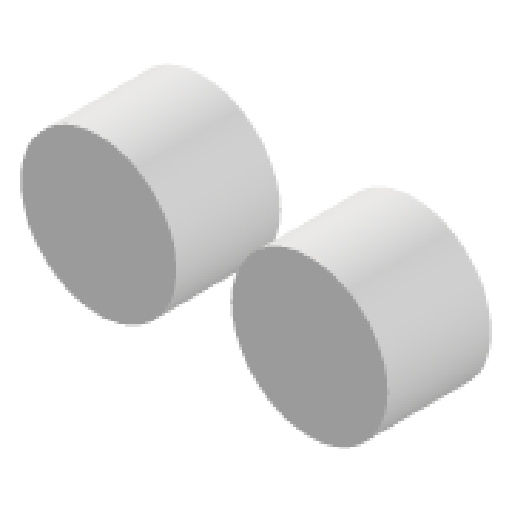
# Autodesk Inventor part: button
Saved by Autodesk Inventor 2026.2 (Build 302298010, 298A)
## iProperties
Created: 2026-04-03
Part Number: button
Material: Generic
Document SubType Name: Modeling
Designer: jocel
Density: 1 g/cm^3
Appearance: Default
Author: jocel
Autodesk Inventor part; units mm, degrees
ref_plane "YZ Plane" through (0, 0, 0) normal (1, 0, 0) x (0, 1, 0)
ref_plane "XZ Plane" through (0, 0, 0) normal (0, 1, 0) x (-1, 0, 0)
ref_plane "XY Plane" through (0, 0, 0) normal (0, 0, 1) x (1, 0, 0)
sketch "Sketch1" plane through (0, 0, 0) normal (0, 0, 1) x (1, 0, 0)
  line L0 (0, 0) -> (-80, 0) projected
  line L1 (0, 0.4115) -> (-80, 0.4115) projected
  circle A0 centre (-65.8472, 0) radius 3
  circle A1 centre (-57.719, 0) radius 3
  dimension "d0" = 6
  dimension "d1" = 6
  constraints: 2 centre point, 2 point on line
  measures "d0" diameter of A0
  measures "d1" diameter of A1
extrude "Extrusion1" add sketch "Sketch1" along normal blind 4 contours A1 L0 | L0 A1 L1 | L1 A1 | A0 L0 | L0 A0 L1 | L1 A0
body "Solid1"
